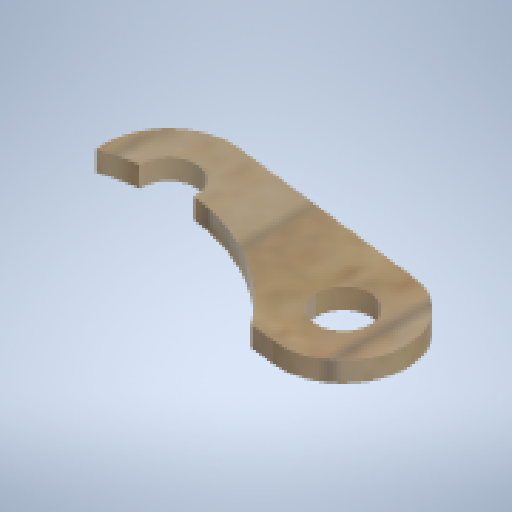
# Autodesk Inventor part: gear_plate_2
Saved by Autodesk Inventor 2026.1 (Build 301233020, 233B)
## iProperties
Created: 2024-04-01
Part Number: gear_plate_2
Material: 木材 (カエデ材)
Document SubType Name: Modeling
Designer: hibik
Density: 0.67 g/cm^3
Appearance: ナチュラル カエデ材 - 光沢 濃い着色
Author: hibik
Autodesk Inventor part; units mm, degrees
ref_plane "YZ Plane" through (0, 0, 0) normal (1, 0, 0) x (0, 1, 0)
ref_plane "XZ Plane" through (0, 0, 0) normal (0, 1, 0) x (-1, 0, 0)
ref_plane "XY Plane" through (0, 0, 0) normal (0, 0, 1) x (1, 0, 0)
sketch "スケッチ1" plane through (0, 0, 0) normal (0, 1, 0) x (-1, 0, 0)
  line L0 (25, 0) -> (-25, 0)
  line L1 (-25, 0) -> (-25, -107)
  line L2 (-25, -107) -> (25, -107)
  line L3 (25, -107) -> (25, 0)
  circle A0 centre (0, 0) radius 25
  circle A1 centre (0, 0) radius 57 construction
  circle A2 centre (0, -82) radius 25
  circle A3 centre (0, 0) radius 75 construction
  circle A4 centre (0, -82) radius 10.75
  circle A5 centre (0, 0) radius 10
  circle A6 centre (0, 0) radius 82
  circle A7 centre (-78.9027, -72.2729) radius 25
  circle A8 centre (-78.9027, -72.2729) radius 10.75
  line L4 (-78.9027, -72.2729) -> (-81.9615, -97.085)
  line L5 (-81.9615, -97.085) -> (-3.0588, -106.8122)
  line L6 (3.0588, -57.1878) -> (-75.8438, -47.4607)
  point P0 (25, -78.0961)
  point P1 (10.7269, -81.2954)
  point P2 (-10.7269, -81.2954)
  point P3 (-25, -78.0961)
  point P4 (-65.9901, -48.6755)
  point P5 (25, -82)
  dimension "d0" = 114
  dimension "d2" = 150
  dimension "d3" = 21.5
  dimension "d4" = 20
  dimension "d5" = 50
  dimension "d13" = 79.5
  constraints: 14 end point, 8 centre point, 8 coincident, 8 tangent, 5 point on circle, 2 equal radius, 2 parallel, 2 perpendicular, 1 horizontal, 1 midpoint, 1 vertical alignment, 4 other
  measures "d0" diameter of A1
  measures "d2" diameter of A3
  measures "d3" diameter of A4
  measures "d4" diameter of A5
  measures "d5" distance of L1.end L2.end
  measures "d13" distance from line of A2.centre L4
extrude "押し出し1" add sketch "スケッチ1" along normal blind 8 contours L3 A2 A6 | A2 A6 A4 | A6 A7 L6 | A6 A2 L1 | L1 L5 A7 A6 | L5 L1 A2 | A7 picked at (-16.5005, -84.9893)
